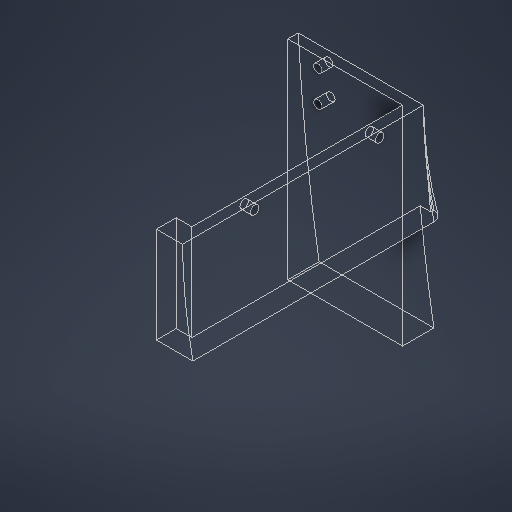
# Autodesk Inventor part: Base Side Armor - Left
Saved by Autodesk Inventor 2026.2 (Build 302298000, 298)
## iProperties
Created: 2024-09-28
Part Number: Base Side Armor - Left
Material: Generic
Document SubType Name: Modeling
Designer: Ethan
Density: 1 g/cm^3
Appearance: Default
Author: Ethan
Autodesk Inventor part; units mm, degrees
ref_plane "Back of Base Plane" through (0, 0, -70.0556) normal (0, 0, 1) x (1, 0, 0)
ref_plane "Side of Base Plane" through (6.5, 0, 0) normal (1, 0, 0) x (0, 1, 0)
ref_plane "Side Bolt Offset Plane" through (16.2, 0, 0) normal (1, 0, 0) x (0, 1, 0)
ref_plane "Back Bolt Offset Plane" through (0, 0, -78.0556) normal (0, 0, 1) x (1, 0, 0)
sketch "Interface - EDIT TO CHANGE SHAPE" plane through (0, 0, 0) normal (0, 1, 0) x (-1, 0, 0)
  line L0 (0, 0) -> (-14, 0) construction
  line L1 (-14, 0) -> (-14, -74.0556) construction
  line L2 (-31, -70.0556) -> (53, -70.0556) construction
  line L3 (-19, -83.0556) -> (41, -83.0556)
  line L4 (0, -106.1556) -> (0, 55.5444) construction
  line L5 (-6.5, -106.1556) -> (-6.5, 55.5444) construction
  line L6 (-14, -76.0556) -> (-14, 22.9444)
  line L7 (-14, 22.9444) -> (-6.5, 22.9444)
  line L8 (-6.5, 22.9444) -> (-6.5, 32.4444)
  line L9 (-6.5, 32.4444) -> (-19, 32.4444)
  line L10 (-19, 32.4444) -> (-19, -83.0556)
  line L11 (-12, -78.0556) -> (41, -78.0556)
  line L12 (41, -78.0556) -> (41, -83.0556)
  line L13 (-14, -76.0556) -> (-14, -78.0556)
  line L14 (-14, -78.0556) -> (-12, -78.0556)
  point P0 (27.5, -70.0556)
  dimension "d11" = 14
  dimension "d65" = 101
  dimension "d66" = 7.5
  dimension "d67" = 9.5
  dimension "d68" = 60
  dimension "d69" = 5
  constraints: 24 end point, 5 horizontal, 5 point on line, 3 vertical, 1 perpendicular
  measures "d11" distance between parallel lines of L1 L4
  measures "d65" distance of L13.end L6.end
  measures "d66" distance of L6.end L7.end
  measures "d67" distance of L7.end L8.end
  measures "d68" distance of L3.start L3.end
  measures "d69" distance between parallel lines of L3 L11
extrude "Interface - EDIT TO CHANGE HEIGHT" add sketch "Interface - EDIT TO CHANGE SHAPE" along normal mid plane 46
sketch "Sketch18" plane through (0, -23, 0) normal (0, -1, 0) x (1, 0, 0)
  line L0 (14, -78.0556) -> (14, 22.9444) projected
  line L1 (14, -78.0556) -> (-41, -78.0556)
  line L2 (-41, -78.0556) -> (-41, -83.0556)
  line L3 (-41, -83.0556) -> (14, -83.0556)
  line L4 (14, -83.0556) -> (14, -78.0556)
  point P0 (0, 0)
  constraints: 8 end point, 2 parallel, 1 horizontal, 1 perpendicular
extrude "Extrusion15" add sketch "Sketch18" along normal blind 54
sketch "Sketch19" plane through (19, 23, -83.0556) normal (0, 0, -1) x (-1, 0, 0)
  line L0 (0, -46) -> (0, 0) projected
  line L1 (0, -46) -> (-5, -46)
  arc A0 (-5, -46) -> (0, 0) centre (-238.4597, 2.6478) ccw
  point P0 (19, -23)
  dimension "d76" = 5
  constraints: 2 end point, 2 point on circle, 1 centre point, 1 horizontal
  measures "d76" distance of L0.start L1.end
extrude "Extrusion16" add sketch "Sketch19" against normal blind 115.5
sketch "Sketch20" plane through (-41, 23, -83.0556) normal (-1, 0, 0) x (0, 0, 1)
  line L0 (0, -100) -> (0, 0) projected
  line L1 (0, -100) -> (-10, -100)
  arc A0 (-10, -100) -> (0, 0) centre (-1100.4358, 59.5436) ccw
  point P0 (83.0556, -23)
  dimension "d79" = 10
  constraints: 2 end point, 2 point on circle, 1 centre point, 1 horizontal
  measures "d79" distance of L0.start L1.end
extrude "Extrusion17" add sketch "Sketch20" against normal blind 60
sketch "Sketch21" plane through (14, -23, -83.0556) normal (0, 0, 1) x (1, 0, 0)
  line L0 (0, 0) -> (5, 0) projected
  line L1 (0, 0) -> (0, -54) projected
  line L2 (5, 0) -> (0, 0)
  line L3 (0, 0) -> (0, -54)
  line L4 (0, -54) -> (5, -54)
  line L5 (5, -54) -> (5, 0)
  point P0 (-14, 23)
  constraints: 8 end point, 2 parallel, 1 horizontal, 1 perpendicular
extrude "Extrusion18" cut sketch "Sketch21" against normal blind 10
sketch "Sketch22" plane through (24, -23, -83.0556) normal (0, 0, -1) x (-1, 0, 0)
  line L0 (5, 0) -> (5, 46) projected
  arc A0 (0, 0) -> (5, 46) centre (-233.4597, 48.6478) ccw projected
  line L1 (5, 0) -> (0, 0) projected
  point P0 (24, 23)
revolve "Revolution3" add sketch "Sketch22" angle 90 about axis through (19, -23, -83.0556) along (0, 1, 0)
sketch "Sketch23" plane through (-41, 23, -78.0556) normal (0, 0, 1) x (1, 0, 0)
  circle A0 centre (14.387, -5) radius 2
  circle A1 centre (14.387, -20) radius 2
  line L0 (55, 0) -> (55, -46) projected
  line L1 (0, 0) -> (55, 0) projected
  point P0 (41, -23)
  dimension "d85" = 4
  dimension "d86" = 4
  dimension "d87" = 40.613
  dimension "d88" = 40.613
  dimension "d89" = 5
  dimension "d93" = 15
  constraints: 2 centre point
  measures "d85" diameter of A1
  measures "d86" diameter of A0
  measures "d87" distance from line of L0 A0.centre
  measures "d88" distance from line of L0 A1.centre
  measures "d89" distance from line of L1 A0.centre
  measures "d93" distance of A0.centre A1.centre
extrude "Extrusion19" cut sketch "Sketch23" against normal blind 10
sketch "Sketch24" plane through (14, -23, 22.9444) normal (-1, 0, 0) x (0, 0, 1)
  circle A0 centre (-85, 43) radius 2
  circle A1 centre (-25, 43) radius 2
  line L0 (-101, 46) -> (0, 46) projected
  line L1 (-101, 0) -> (-101, 46) projected
  point P0 (-22.9444, 23)
  dimension "d94" = 4
  dimension "d95" = 4
  dimension "d96" = 60
  dimension "d97" = 3
  dimension "d98" = 3
  dimension "d99" = 16
  constraints: 2 centre point
  measures "d94" diameter of A1
  measures "d95" diameter of A0
  measures "d96" distance of A1.centre A0.centre
  measures "d97" distance from line of L0 A0.centre
  measures "d98" distance from line of L0 A1.centre
  measures "d99" distance from line of L1 A0.centre
extrude "Extrusion20" cut sketch "Sketch24" against normal blind 10
equation "\"d88\" = d87"
equation "\"d95\" = d94"
body "Solid2"
